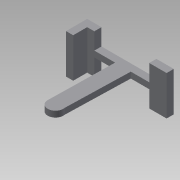
# Autodesk Inventor part: cover sepatu32
Saved by Autodesk Inventor 2015 SP1 (Build 190203100, 203)
## iProperties
Created: 2015-04-15
Part Number: cover sepatu32
Material: Generic
Document SubType Name: Modeling
Designer: Rafi Kurnia Putra
Density: 1 g/cm^3
Appearance: Default
Author: Rafi Kurnia Putra
Autodesk Inventor part; units mm, degrees
ref_plane "YZ Plane" through (0, 0, 0) normal (1, 0, 0) x (0, 1, 0)
ref_plane "Work Plane5" through (0, 0, 9.5) normal (0, 0, 1) x (1, 0, 0)
sketch "Sketch4" plane through (0, 0, 9.5) normal (0, 0, 1) x (1, 0, 0)
  arc A0 (-3.3085, -7.69) -> (3.0707, -6.4871) centre (-0.1029, -7.1736) ccw
  line L0 (3.0707, -6.4871) -> (3.7901, 20.5)
  line L1 (-2.7798, 20.5) -> (-3.3085, -7.69)
  line L2 (-3.8298, 20.5) -> (-2.7798, 20.5)
  line L3 (3.7901, 20.5) -> (4.8401, 20.5)
  line L4 (-11.5, 20.5) -> (-12.5, 20.5) projected
  line L5 (11.5, 20.5) -> (9.5, 20.5) projected
  line L6 (-12.5, 20.5) -> (-2.7798, 20.5)
  line L7 (3.7901, 20.5) -> (18.7901, 20.5)
  line L8 (-12.5, 20.5) -> (-12.5, 14.637)
  line L9 (-12.5, 14.637) -> (-12.5, 20.5)
  line L10 (-12.5, 14.637) -> (-14.5, 14.637)
  line L11 (-14.5, 14.637) -> (-14.5, 22.5)
  line L12 (-14.5, 22.5) -> (18.7901, 22.5)
  line L13 (18.7901, 22.5) -> (18.7901, 20.5)
  line L14 (-2.7798, 20.5) -> (3.7901, 20.5)
  point P0 (0, 0)
  point P1 (-0.3189, -10.4133)
  dimension "d34" = 15
  dimension "d36" = 2
  dimension "d52" = 2
  constraints: 26 end point, 3 perpendicular, 3 point on circle, 2 horizontal, 1 centre point, 1 collinear, 1 point on line, 2 other
  measures "d34" distance of L0.end L7.end
  measures "d36" distance of L8.end L10.end
  measures "d52" distance between parallel lines of L6 L12
extrude "Extrusion7" add sketch "Sketch4" along normal mid plane 2.5 contours L1 L14 L0 A0
extrude "Extrusion8" add sketch "Sketch4" along normal mid plane 17 contours L2 L6 L4 L8 L10 L11 L12 L13 L7 L5 L3 L14
ref_plane "Work Plane4" through (-12.5, 22.5, 0) normal (0, 1, 0) x (1, 0, 0)
sketch "Sketch5" plane through (-12.5, 22.5, 0) normal (0, 1, 0) x (1, 0, 0)
  line L0 (-2, -11.5) -> (27, -11.5)
  line L1 (27, -11.5) -> (27, -7.5)
  line L2 (27, -7.5) -> (-2, -7.5)
  line L3 (-2, -7.5) -> (-2, -11.5)
  line L4 (15.5, -9.5) -> (9.5, -9.5) projected
  line L5 (-2, -11.5) -> (27, -7.5) construction
  line L6 (27, -11.5) -> (-2, -7.5) construction
  line L7 (0, -1) -> (25, -1)
  line L8 (25, -1) -> (25, -7.5)
  line L9 (25, -7.5) -> (0, -7.5)
  line L10 (0, -7.5) -> (0, -1)
  line L11 (0, -9.5) -> (0, -18) projected
  line L12 (0, -18) -> (31.2901, -18) projected
  line L13 (0, -11.5) -> (25, -11.5)
  line L14 (25, -11.5) -> (25, -18)
  line L15 (25, -18) -> (0, -18)
  line L16 (0, -18) -> (0, -11.5)
  point P0 (12.5, 0)
  point P1 (12.5, -9.5)
  constraints: 28 end point, 6 parallel, 4 point on line, 3 horizontal, 3 midpoint, 3 perpendicular
extrude "Extrusion9" cut sketch "Sketch5" against normal through all contours L0 L14 L12 L11 | L10 L7 L8 L2
sketch "Sketch6" plane through (-14.5, 22.5, 1) normal (0, 1, 0) x (1, 0, 0)
  line L0 (2, -6.5) -> (27, -6.5) projected
  line L1 (2, 0) -> (4, 0)
  line L2 (4, 0) -> (4, -6.5)
  line L3 (4, -6.5) -> (2, -6.5)
  line L4 (2, -6.5) -> (2, 0)
  line L5 (27, -10.5) -> (2, -10.5) projected
  line L6 (2, -17) -> (4, -17)
  line L7 (4, -17) -> (4, -10.5)
  line L8 (4, -10.5) -> (2, -10.5)
  line L9 (2, -10.5) -> (2, -17)
  line L10 (27, 0) -> (25, 0)
  line L11 (25, 0) -> (25, -6.5)
  line L12 (25, -6.5) -> (27, -6.5)
  line L13 (27, -6.5) -> (27, 0)
  line L14 (27, -10.5) -> (25, -10.5)
  line L15 (25, -10.5) -> (25, -17)
  line L16 (25, -17) -> (27, -17)
  line L17 (27, -17) -> (27, -10.5)
  point P0 (14.5, 1)
  dimension "d43" = 2
  dimension "d44" = 2
  dimension "d45" = 2
  dimension "d46" = 2
  constraints: 32 end point, 8 parallel, 4 horizontal, 4 perpendicular, 4 point on line
  measures "d43" distance of L2.end L3.end
  measures "d44" distance of L8.end L7.end
  measures "d45" distance of L12.end L11.end
  measures "d46" distance of L16.end L15.end
extrude "Extrusion10" add sketch "Sketch6" along normal mid plane 4
sketch "Sketch7" plane through (18.7901, 22.5, 18) normal (0, 1, 0) x (1, 0, 0)
  line L0 (-8.2901, 0) -> (0, 0) projected
  line L1 (0, 17) -> (5, 17)
  line L2 (5, 17) -> (5, 0)
  line L3 (5, 0) -> (0, 0)
  line L4 (0, 0) -> (0, 17)
  point P0 (-18.7901, 18)
  dimension "d49" = 5
  constraints: 8 end point, 2 parallel, 1 horizontal, 1 perpendicular, 1 point on line
  measures "d49" distance of L3.end L2.end
extrude "Extrusion11" cut sketch "Sketch7" against normal through all
sketch "Sketch8" plane through (0, 0, 18) normal (0, 0, 1) x (1, 0, 0)
  line L0 (12.5, 24.5) -> (18.7901, 24.5)
  line L1 (18.7901, 24.5) -> (18.7901, 22.5)
  line L2 (18.7901, 22.5) -> (12.5, 22.5)
  line L3 (12.5, 22.5) -> (12.5, 24.5)
  line L4 (-12.5, 24.5) -> (-14.5, 24.5)
  line L5 (-14.5, 24.5) -> (-14.5, 22.5)
  line L6 (-14.5, 22.5) -> (-12.5, 22.5)
  line L7 (-12.5, 22.5) -> (-12.5, 24.5)
  point P0 (0, 0)
  constraints: 16 end point, 4 parallel, 2 horizontal, 2 perpendicular
extrude "Extrusion12" add sketch "Sketch8" against normal blind 17
sketch "Sketch9" plane through (-10.5, 22.5, 11.5) normal (0, 1, 0) x (1, 0, 0)
  line L0 (0, 0) -> (0, 4)
  line L1 (21, 0) -> (21, 4)
  line L2 (23, 0) -> (21, 0) projected
  line L3 (23, 0) -> (23, 4) projected
  line L4 (21, 4) -> (23, 4) projected
  line L5 (-2, 4) -> (0, 4) projected
  line L6 (-2, 0) -> (-2, 4) projected
  line L7 (0, 0) -> (-2, 0) projected
  point P0 (10.5, 11.5)
  constraints: 4 end point, 2 vertical
extrude "Extrusion13" add sketch "Sketch9" along normal blind 2
sketch "Sketch10" plane through (-10.5, 20.5, 11.5) normal (0, 0, 1) x (1, 0, 0)
  line L0 (0, 4) -> (21, 4)
  line L1 (21, 4) -> (21, 2)
  line L2 (21, 2) -> (0, 2)
  line L3 (0, 2) -> (0, 4)
  point P0 (10.5, -20.5)
  constraints: 8 end point, 2 parallel, 1 horizontal, 1 perpendicular
extrude "Extrusion14" add sketch "Sketch10" against normal blind 4
sketch "Sketch12" plane through (0, 0, 18) normal (0, 0, 1) x (1, 0, 0)
  line L0 (18.7901, 24.5) -> (18.7901, 20.5) projected
  line L1 (-14.5, 24.5) -> (18.7901, 24.5)
  line L2 (18.7901, 24.5) -> (18.7901, 23.5)
  line L3 (18.7901, 23.5) -> (-14.5, 23.5)
  line L4 (-14.5, 23.5) -> (-14.5, 24.5)
  point P0 (0, 0)
  dimension "d59" = 1
  constraints: 8 end point, 2 parallel, 1 horizontal, 1 perpendicular, 1 point on line
  measures "d59" distance of L1.end L2.end
extrude "Extrusion15" cut sketch "Sketch12" against normal through all
sketch "Sketch13" plane through (0, 0, 18) normal (0, 0, 1) x (1, 0, 0)
  line L0 (-14.5, 23.5) -> (-15.5, 23.5)
  line L1 (-15.5, 23.5) -> (-15.5, 14.637)
  line L2 (-15.5, 14.637) -> (-14.5, 14.637)
  line L3 (-14.5, 14.637) -> (-14.5, 23.5)
  point P0 (0, 0)
  dimension "d62" = 1
  constraints: 8 end point, 2 parallel, 1 horizontal, 1 perpendicular
  measures "d62" distance of L2.end L1.end
extrude "Extrusion16" add sketch "Sketch13" against normal blind 17
sketch "Sketch15" plane through (10.5, 23.5, 18) normal (0, 1, 0) x (1, 0, 0)
  line L0 (0, 17) -> (3, 17)
  line L1 (3, 17) -> (3, 10.5)
  line L2 (3, 10.5) -> (0, 10.5)
  line L3 (0, 10.5) -> (0, 17)
  line L4 (0, 0) -> (3, 0)
  line L5 (3, 0) -> (3, 6.4739)
  line L6 (3, 6.4739) -> (0, 6.4739)
  line L7 (0, 6.4739) -> (0, 0)
  point P0 (-10.5, 18)
  dimension "d70" = 3
  constraints: 16 end point, 4 parallel, 2 horizontal, 2 perpendicular, 1 point on line
  measures "d70" distance of L0.start L0.end
extrude "Extrusion18" cut sketch "Sketch15" against normal up to next
sketch "Sketch16" plane through (-10.5, 23.5, 11.5) normal (0, 1, 0) x (1, 0, 0)
  line L0 (0, 10.5) -> (1, 10.5)
  line L1 (1, 10.5) -> (1, -6.5)
  line L2 (1, -6.5) -> (0, -6.5)
  line L3 (0, -6.5) -> (0, 10.5)
  point P0 (10.5, 11.5)
  constraints: 8 end point, 2 parallel, 1 horizontal, 1 perpendicular
extrude "Extrusion19" add sketch "Sketch16" against normal blind 3
sketch "Sketch17" plane through (-12.5, 14.637, 18) normal (1, 0, 0) x (0, 0, -1)
  line L0 (17, 5.863) -> (0, 5.863) projected
  line L1 (0, 0) -> (0, 5.863) projected
  line L2 (17, 0) -> (0, 0) projected
  line L3 (17, 5.863) -> (17, 0) projected
  point P0 (18, -14.637)
extrude "Extrusion20" cut sketch "Sketch17" against normal blind 2
sketch "Sketch18" plane through (-15.5, 14.637, 18) normal (-1, 0, 0) x (0, 0, 1)
  line L0 (0, 5.863) -> (-17, 5.863) projected
  line L1 (0, 8.863) -> (0, 0) projected
  line L2 (0, 8.863) -> (-17, 8.863) projected
  line L3 (-17, 0) -> (-17, 8.863) projected
  line L4 (0, 0) -> (-17, 0) projected
  point P0 (-18, -14.637)
extrude "Extrusion21" add sketch "Sketch18" along normal blind 2
sketch "Sketch19" plane through (18.7901, 23.5, 18) normal (0, 1, 0) x (1, 0, 0)
  line L0 (-28.2901, 17) -> (-30.2901, 17)
  line L1 (-30.2901, 17) -> (-30.2901, 10.5)
  line L2 (-30.2901, 10.5) -> (-28.2901, 10.5)
  line L3 (-28.2901, 10.5) -> (-28.2901, 17)
  line L4 (-28.2901, 0) -> (-36.2901, 0) projected
  line L5 (-28.2901, 6.5) -> (-30.2901, 6.5)
  line L6 (-30.2901, 6.5) -> (-30.2901, 0)
  line L7 (-30.2901, 0) -> (-28.2901, 0)
  line L8 (-28.2901, 0) -> (-28.2901, 6.5)
  line L9 (-5.2901, 17) -> (-7.2901, 17)
  line L10 (-7.2901, 17) -> (-7.2901, 0)
  line L11 (-7.2901, 0) -> (-5.2901, 0)
  line L12 (-5.2901, 0) -> (-5.2901, 17)
  point P0 (-18.7901, 18)
  dimension "d77" = 2
  dimension "d78" = 2
  constraints: 24 end point, 6 parallel, 3 horizontal, 3 perpendicular, 3 point on line
  measures "d77" distance of L2.end L1.end
  measures "d78" distance of L11.end L10.end
extrude "Extrusion22" cut sketch "Sketch19" against normal up to next contours L3 L2 L1 L0 | L4 L6 L5 L8
extrude "Extrusion23" add sketch "Sketch19" against normal blind 3 contours L12 L11 L10 L9
sketch "Sketch20" plane through (18.7901, 20.5, 1) normal (0, -1, 0) x (1, 0, 0)
  line L0 (-22.0985, 7.25) -> (-15.646, 7.25) projected
  line L1 (-15.646, 9.75) -> (-22.0985, 9.75) projected
  line L2 (-7.2901, 17) -> (-7.2901, 10.5261) projected
  line L3 (-30.2901, 17) -> (-30.2901, 10.5) projected
  line L4 (-30.2901, 13) -> (-7.2901, 13)
  line L5 (-7.2901, 13) -> (-7.2901, 9.75)
  line L6 (-7.2901, 9.75) -> (-30.2901, 9.75)
  line L7 (-30.2901, 9.75) -> (-30.2901, 13)
  line L8 (-30.2901, 4) -> (-7.2901, 4)
  line L9 (-7.2901, 4) -> (-7.2901, 7.25)
  line L10 (-7.2901, 7.25) -> (-30.2901, 7.25)
  line L11 (-30.2901, 7.25) -> (-30.2901, 4)
  point P0 (-18.7901, -1)
  point P1 (-15.7194, 7.25)
  point P2 (-15.7194, 9.75)
  constraints: 16 end point, 4 parallel, 3 point on line, 2 horizontal, 2 perpendicular
extrude "Extrusion24" cut sketch "Sketch20" against normal through all
sketch "Sketch21" plane through (18.7901, 23.5, 18) normal (0, 1, 0) x (1, 0, 0)
  line L0 (0, 17) -> (0, 0) projected
  line L1 (-36.2901, 17) -> (0, 17)
  line L2 (0, 17) -> (0, 16.75)
  line L3 (0, 16.75) -> (-36.2901, 16.75)
  line L4 (-36.2901, 16.75) -> (-36.2901, 17)
  line L5 (-36.2901, 0) -> (-36.2901, 17) projected
  line L6 (0, 0) -> (-36.2901, 0)
  line L7 (-36.2901, 0) -> (-36.2901, 0.25)
  line L8 (-36.2901, 0.25) -> (0, 0.25)
  line L9 (0, 0.25) -> (0, 0)
  point P0 (-18.7901, 18)
  dimension "d85" = 0.25
  dimension "d86" = 0.25
  constraints: 16 end point, 4 parallel, 2 horizontal, 2 perpendicular, 2 point on line
  measures "d85" distance of L1.end L2.end
  measures "d86" distance of L6.end L7.end
extrude "Extrusion25" cut sketch "Sketch21" against normal through all contours L0 L3 L4 L1 | L0 L6 L5 L8
body "Solid1"
